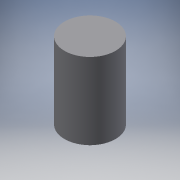
# Autodesk Inventor part: Motor
Saved by Autodesk Inventor 2019 (Build 230136000, 136)
## iProperties
Created: 2019-03-05
Part Number: Motor
Material: Generic
Document SubType Name: Modeling
Designer: alarr
Density: 1 g/cm^3
Appearance: Default
Author: alarr
Autodesk Inventor part; units mm, degrees
ref_plane "YZ Plane" through (0, 0, 0) normal (1, 0, 0) x (0, 1, 0)
ref_plane "XZ Plane" through (0, 0, 0) normal (0, 1, 0) x (-1, 0, 0)
ref_plane "XY Plane" through (0, 0, 0) normal (0, 0, 1) x (1, 0, 0)
sketch "Sketch1" plane through (0, 0, 0) normal (0, 1, 0) x (-1, 0, 0)
  circle A0 centre (0, 0) radius 6.5405
  dimension "d0" = 13.081
  constraints: 1 centre point, 1 coincident
  measures "d0" diameter of A0
extrude "Extrusion1" add sketch "Sketch1" along normal blind 3.683
sketch "Sketch2" plane through (0, 3.683, 0) normal (0, 1, 0) x (1, 0, 0)
  circle A0 centre (0, 0) radius 19.05
  dimension "d3" = 38.1
  constraints: 1 centre point, 1 coincident
  measures "d3" diameter of A0
extrude "Extrusion2" add sketch "Sketch2" along normal blind 57.15
sketch "Sketch3" plane through (0, 0, 0) normal (0, -1, 0) x (1, 0, 0)
  circle A0 centre (0, 0) radius 1.5875
  dimension "d6" = 3.175
  constraints: 1 centre point, 1 coincident
  measures "d6" diameter of A0
extrude "Extrusion3" add sketch "Sketch3" along normal blind 8.89
sketch "Sketch4" plane through (0, 3.683, 0) normal (0, -1, 0) x (1, 0, 0)
  circle A0 centre (0, 0) radius 19.05 projected
  circle A1 centre (0, 0) radius 12.7 construction
  circle A2 centre (0, 0) radius 1.5875 projected
  line L0 (0, 0) -> (0, -12.7) construction
  line L1 (0, 0) -> (-12.7, 0) construction
  line L2 (0, 0) -> (12.7, 0) construction
  circle A3 centre (0, -12.7) radius 1.27
  circle A4 centre (-12.7, 0) radius 1.27
  circle A5 centre (12.7, 0) radius 1.27
  dimension "d9" = 25.4
  dimension "d10" = 2.54
  constraints: 6 end point, 4 centre point, 4 coincident, 3 point on circle, 2 equal radius, 1 perpendicular, 1 point on line, 1 vertical
  measures "d9" diameter of A1
  measures "d10" diameter of A3
extrude "Extrusion4" cut sketch "Sketch4" against normal blind 2.54 contours A3 | A4 | A5
body "Solid1"
